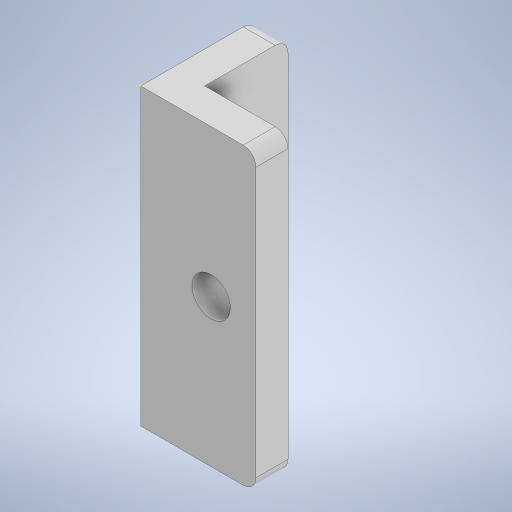
# Autodesk Inventor part: pieza 1-20
Saved by Autodesk Inventor 2024.2 (Build 282272000, 272)
## iProperties
Created: 2024-10-10
Part Number: pieza 1-20
Material: Generic
Document SubType Name: Modeling
Designer: Precisión-18
Density: 1 g/cm^3
Appearance: Default
Author: Precisión-18
Autodesk Inventor part; units mm, degrees
ref_plane "YZ Plane" through (0, 0, 0) normal (1, 0, 0) x (0, 1, 0)
ref_plane "XZ Plane" through (0, 0, 0) normal (0, 1, 0) x (-1, 0, 0)
ref_plane "XY Plane" through (0, 0, 0) normal (0, 0, 1) x (1, 0, 0)
sketch "Sketch1" plane through (0, 0, 0) normal (0, 0, 1) x (1, 0, 0)
  point P0 (0, 0)
sketch "Sketch2" plane through (0, 0, 0) normal (0, 1, 0) x (-1, 0, 0)
  line L0 (0, 0) -> (0, -9)
  line L1 (0, -9) -> (-2.5, -9)
  line L2 (-2.5, -9) -> (-2.5, -2.5)
  line L3 (-2.5, -2.5) -> (-9, -2.5)
  line L4 (-9, -2.5) -> (-9, 0)
  line L5 (-9, 0) -> (0, 0)
  dimension "d0" = 9
  dimension "d1" = 2.5
  dimension "d2" = 9
  dimension "d3" = 2.5
  constraints: 12 end point, 5 perpendicular, 1 vertical
  measures "d0" distance of L0.start L0.end
  measures "d1" distance of L0.end L1.end
  measures "d2" distance of L4.end L0.start
  measures "d3" distance of L3.end L4.end
extrude "Extrusion1" add sketch "Sketch2" against normal blind 23
sketch "Sketch3" plane through (0, 0, 0) normal (0, 0, 1) x (1, 0, 0)
  circle A0 centre (5.5, -11.5) radius 1.5
  line L0 (0, 0) -> (9, 0) projected
  line L1 (0, 0) -> (0, -23) projected
  dimension "d6" = 3
  dimension "d7" = 11.5
  dimension "d8" = 5.5
  constraints: 1 centre point
  measures "d6" diameter of A0
  measures "d7" distance from line of A0.centre L0
  measures "d8" distance from line of L1 A0.centre
extrude "Extrusion2" cut sketch "Sketch3" against normal blind 23
sketch "Sketch4" plane through (0, 0, -9) normal (-1, 0, 0) x (0, 0, 1)
  circle A0 centre (3.5, -5.5) radius 1.5
  circle A1 centre (3.5, -17.5) radius 1.5
  line L0 (0, 0) -> (9, 0) projected
  line L1 (9, -23) -> (0, -23) projected
  line L2 (9, 0) -> (9, -23) projected
  dimension "d11" = 3
  dimension "d12" = 3
  dimension "d13" = 5.5
  dimension "d14" = 5.5
  dimension "d15" = 12
  dimension "d16" = 5.5
  constraints: 2 centre point
  measures "d11" diameter of A1
  measures "d12" diameter of A0
  measures "d13" distance from line of L0 A0.centre
  measures "d14" distance from line of L1 A1.centre
  measures "d15" distance of A1.centre A0.centre
  measures "d16" distance from line of A0.centre L2
extrude "Extrusion3" cut sketch "Sketch4" against normal blind 23
fillet "Fillet1" radius 1 4 edges at (1.25, 0, -9) (9, 0, -1.25) (9, -23, -1.25) (1.25, -23, -9)
body "Solid1"
